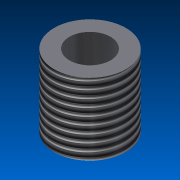
# Autodesk Inventor part: 12mm Incremental Encoder Threaded Tube
Saved by Autodesk Inventor 2014 (Build 180170000, 170)
## iProperties
Created: 2011-11-07
Part Number: 12mm Incremental Encoder Threaded Tube
Document SubType Name: Modeling
Designer: sdarley
Density: 1 g/cm^3
Material: Generic
Appearance: Steel - Polished
Author: sdarley
Autodesk Inventor part; units mm, degrees
ref_plane "YZ Plane" through (0, 0, 0) normal (1, 0, 0) x (0, 1, 0)
ref_plane "XZ Plane" through (0, 0, 0) normal (0, 1, 0) x (-1, 0, 0)
ref_plane "XY Plane" through (0, 0, 0) normal (0, 0, 1) x (1, 0, 0)
sketch "Sketch1" plane through (0, 0, 0) normal (0, 0, 1) x (1, 0, 0)
  line L0 (0, 4.5) -> (0, -4.5) projected
  line L1 (-0.25, 4.5) -> (0, 4.5) projected
  line L2 (-0.25, 5) -> (-0.25, 4.5) projected
  arc A0 (-0.25, 5) -> (-1.25, 6) centre (-1.25, 5) ccw projected
  line L3 (-11.6, 6) -> (-1.25, 6) projected
  arc A1 (-11.6, 6) -> (-12.6, 5) centre (-11.6, 5) ccw projected
  line L4 (-12.6, 4.5) -> (-12.6, 5) projected
  line L5 (-12.85, 4.5) -> (-12.6, 4.5) projected
  line L6 (-12.85, -4.5) -> (-12.85, 4.5) projected
  line L7 (-12.6, -4.5) -> (-12.85, -4.5) projected
  line L8 (-12.6, -5) -> (-12.6, -4.5) projected
  arc A2 (-12.6, -5) -> (-11.6, -6) centre (-11.6, -5) ccw projected
  line L9 (-1.25, -6) -> (-11.6, -6) projected
  arc A3 (-1.25, -6) -> (-0.25, -5) centre (-1.25, -5) ccw projected
  line L10 (-0.25, -4.5) -> (-0.25, -5) projected
  line L11 (0, -4.5) -> (-0.25, -4.5) projected
  circle A4 centre (-6.425, 0) radius 3.5
  circle A5 centre (-6.425, 0) radius 2
  point P0 (0, 0)
  dimension "d0" = 7
  dimension "d1" = 4
  constraints: 2 centre point, 1 coincident
  measures "d0" diameter of A4
  measures "d1" diameter of A5
extrude "Extrusion1" add sketch "Sketch1" along normal blind 7 contours A4
thread "Thread1" size "M7x0.75" class "6g" standard "ISO Metric profile" full length
body "Solid1"
